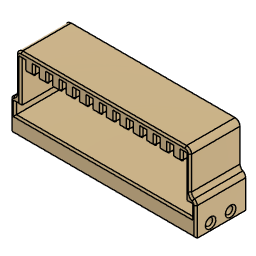
Suporte calha muitos watts 2 v3 (Autodesk Fusion 360 design; units mm, degrees)
Autodesk Fusion 360 part; units mm, degrees
sketch "Sketch1" plane through (0, 0, 0) normal (0, 1, 0) x (1, 0, 0)
  line L0 (0, 0) -> (105, 0)
  line L1 (105, 0) -> (105, -6)
  line L2 (0, -6) -> (0, 0)
  line L3 (51.7, -6) -> (51.7, -31.6)
  line L4 (51.7, -31.6) -> (53.3, -31.6)
  line L5 (53.3, -31.6) -> (53.3, -6)
  line L6 (52.5, -31.6) -> (52.5, 0) construction
  line L7 (3.4, -6) -> (3.4, -31.6)
  line L8 (3.4, -31.6) -> (5, -31.6)
  line L9 (5, -31.6) -> (5, -6)
  line L10 (11.45, -6) -> (11.45, -31.6)
  line L11 (11.45, -31.6) -> (13.05, -31.6)
  line L12 (13.05, -31.6) -> (13.05, -6)
  line L13 (19.5, -6) -> (19.5, -31.6)
  line L14 (19.5, -31.6) -> (21.1, -31.6)
  line L15 (21.1, -31.6) -> (21.1, -6)
  line L16 (27.55, -6) -> (27.55, -31.6)
  line L17 (27.55, -31.6) -> (29.15, -31.6)
  line L18 (29.15, -31.6) -> (29.15, -6)
  line L19 (35.6, -6) -> (35.6, -31.6)
  line L20 (35.6, -31.6) -> (37.2, -31.6)
  line L21 (37.2, -31.6) -> (37.2, -6)
  line L22 (43.65, -6) -> (43.65, -31.6)
  line L23 (43.65, -31.6) -> (45.25, -31.6)
  line L24 (45.25, -31.6) -> (45.25, -6)
  line L25 (59.75, -6) -> (59.75, -31.6)
  line L26 (59.75, -31.6) -> (61.35, -31.6)
  line L27 (61.35, -31.6) -> (61.35, -6)
  line L28 (67.8, -6) -> (67.8, -31.6)
  line L29 (67.8, -31.6) -> (69.4, -31.6)
  line L30 (69.4, -31.6) -> (69.4, -6)
  line L31 (75.85, -6) -> (75.85, -31.6)
  line L32 (75.85, -31.6) -> (77.45, -31.6)
  line L33 (77.45, -31.6) -> (77.45, -6)
  line L34 (83.9, -6) -> (83.9, -31.6)
  line L35 (83.9, -31.6) -> (85.5, -31.6)
  line L36 (85.5, -31.6) -> (85.5, -6)
  line L37 (91.95, -6) -> (91.95, -31.6)
  line L38 (91.95, -31.6) -> (93.55, -31.6)
  line L39 (93.55, -31.6) -> (93.55, -6)
  line L40 (100, -6) -> (100, -31.6)
  line L41 (100, -31.6) -> (101.6, -31.6)
  line L42 (101.6, -31.6) -> (101.6, -6)
  line L43 (11.45, -6) -> (5, -6)
  line L44 (19.5, -6) -> (13.05, -6)
  line L45 (27.55, -6) -> (21.1, -6)
  line L46 (35.6, -6) -> (29.15, -6)
  line L47 (51.7, -6) -> (45.25, -6)
  line L48 (43.65, -6) -> (37.2, -6)
  line L49 (3.4, -6) -> (0, -6)
  line L50 (59.75, -6) -> (53.3, -6)
  line L51 (67.8, -6) -> (61.35, -6)
  line L52 (105, -6) -> (101.6, -6)
  line L53 (100, -6) -> (93.55, -6)
  line L54 (83.9, -6) -> (77.45, -6)
  line L55 (91.95, -6) -> (85.5, -6)
  line L56 (75.85, -6) -> (69.4, -6)
  line L57 (21.4, -31.9) -> (21.4, -6.3)
  line L58 (27.25, -6.3) -> (21.4, -6.3)
  line L59 (27.25, -6.3) -> (27.25, -31.9)
  line L60 (27.25, -31.9) -> (29.45, -31.9)
  line L61 (29.45, -31.9) -> (29.45, -6.3)
  line L62 (35.3, -6.3) -> (29.45, -6.3)
  line L63 (35.3, -6.3) -> (35.3, -31.9)
  line L64 (35.3, -31.9) -> (37.5, -31.9)
  line L65 (37.5, -31.9) -> (37.5, -6.3)
  line L66 (43.35, -6.3) -> (37.5, -6.3)
  line L67 (43.35, -6.3) -> (43.35, -31.9)
  line L68 (43.35, -31.9) -> (45.55, -31.9)
  line L69 (45.55, -31.9) -> (45.55, -6.3)
  line L70 (51.4, -6.3) -> (45.55, -6.3)
  line L71 (51.4, -6.3) -> (51.4, -31.9)
  line L72 (51.4, -31.9) -> (53.6, -31.9)
  line L73 (53.6, -31.9) -> (53.6, -6.3)
  line L74 (59.45, -6.3) -> (53.6, -6.3)
  line L75 (59.45, -6.3) -> (59.45, -31.9)
  line L76 (59.45, -31.9) -> (61.65, -31.9)
  line L77 (61.65, -31.9) -> (61.65, -6.3)
  line L78 (67.5, -6.3) -> (61.65, -6.3)
  line L79 (67.5, -6.3) -> (67.5, -31.9)
  line L80 (67.5, -31.9) -> (69.7, -31.9)
  line L81 (69.7, -31.9) -> (69.7, -6.3)
  line L82 (75.55, -6.3) -> (69.7, -6.3)
  line L83 (75.55, -6.3) -> (75.55, -31.9)
  line L84 (75.55, -31.9) -> (77.75, -31.9)
  line L85 (77.75, -31.9) -> (77.75, -6.3)
  line L86 (83.6, -6.3) -> (77.75, -6.3)
  line L87 (83.6, -6.3) -> (83.6, -31.9)
  line L88 (83.6, -31.9) -> (85.8, -31.9)
  line L89 (85.8, -31.9) -> (85.8, -6.3)
  line L90 (91.65, -6.3) -> (85.8, -6.3)
  line L91 (91.65, -6.3) -> (91.65, -31.9)
  line L92 (91.65, -31.9) -> (93.85, -31.9)
  line L93 (93.85, -31.9) -> (93.85, -6.3)
  line L94 (99.7, -6.3) -> (93.85, -6.3)
  line L95 (99.7, -6.3) -> (99.7, -31.9)
  line L96 (99.7, -31.9) -> (101.9, -31.9)
  line L97 (101.9, -31.9) -> (101.9, -6.3)
  line L98 (105.3, -6.3) -> (101.9, -6.3)
  line L99 (105.3, 0.3) -> (105.3, -6.3)
  line L100 (-0.3, 0.3) -> (105.3, 0.3)
  line L101 (-0.3, -6.3) -> (-0.3, 0.3)
  line L102 (3.1, -6.3) -> (-0.3, -6.3)
  line L103 (3.1, -6.3) -> (3.1, -31.9)
  line L104 (3.1, -31.9) -> (5.3, -31.9)
  line L105 (5.3, -31.9) -> (5.3, -6.3)
  line L106 (11.15, -6.3) -> (5.3, -6.3)
  line L107 (11.15, -6.3) -> (11.15, -31.9)
  line L108 (11.15, -31.9) -> (13.35, -31.9)
  line L109 (13.35, -31.9) -> (13.35, -6.3)
  line L110 (19.2, -6.3) -> (13.35, -6.3)
  line L111 (19.2, -6.3) -> (19.2, -31.9)
  line L112 (19.2, -31.9) -> (21.4, -31.9)
  line L113 (32.15, -34.6) -> (32.15, -9)
  line L114 (32.6, -9) -> (32.15, -9)
  line L115 (32.6, -9) -> (32.6, -34.6)
  line L116 (32.6, -34.6) -> (40.2, -34.6)
  line L117 (40.2, -34.6) -> (40.2, -9)
  line L118 (40.65, -9) -> (40.2, -9)
  line L119 (40.65, -9) -> (40.65, -34.6)
  line L120 (40.65, -34.6) -> (48.25, -34.6)
  line L121 (48.25, -34.6) -> (48.25, -9)
  line L122 (48.7, -9) -> (48.25, -9)
  line L123 (48.7, -9) -> (48.7, -34.6)
  line L124 (48.7, -34.6) -> (56.3, -34.6)
  line L125 (56.3, -34.6) -> (56.3, -9)
  line L126 (56.75, -9) -> (56.3, -9)
  line L127 (56.75, -9) -> (56.75, -34.6)
  line L128 (56.75, -34.6) -> (64.35, -34.6)
  line L129 (64.35, -34.6) -> (64.35, -9)
  line L130 (64.8, -9) -> (64.35, -9)
  line L131 (64.8, -9) -> (64.8, -34.6)
  line L132 (64.8, -34.6) -> (72.4, -34.6)
  line L133 (72.4, -34.6) -> (72.4, -9)
  line L134 (72.85, -9) -> (72.4, -9)
  line L135 (72.85, -9) -> (72.85, -34.6)
  line L136 (72.85, -34.6) -> (80.45, -34.6)
  line L137 (80.45, -34.6) -> (80.45, -9)
  line L138 (80.9, -9) -> (80.45, -9)
  line L139 (80.9, -9) -> (80.9, -34.6)
  line L140 (80.9, -34.6) -> (88.5, -34.6)
  line L141 (88.5, -34.6) -> (88.5, -9)
  line L142 (88.95, -9) -> (88.5, -9)
  line L143 (88.95, -9) -> (88.95, -34.6)
  line L144 (88.95, -34.6) -> (96.55, -34.6)
  line L145 (96.55, -34.6) -> (96.55, -9)
  line L146 (97, -9) -> (96.55, -9)
  line L147 (97, -9) -> (97, -34.6)
  line L148 (97, -34.6) -> (104.6, -34.6)
  line L149 (104.6, -34.6) -> (104.6, -9)
  line L150 (108, -9) -> (104.6, -9)
  line L151 (108, 3) -> (108, -9)
  line L152 (-3, 3) -> (108, 3)
  line L153 (-3, -9) -> (-3, 3)
  line L154 (0.4, -9) -> (-3, -9)
  line L155 (0.4, -9) -> (0.4, -34.6)
  line L156 (0.4, -34.6) -> (8, -34.6)
  line L157 (8, -34.6) -> (8, -9)
  line L158 (8.45, -9) -> (8, -9)
  line L159 (8.45, -9) -> (8.45, -34.6)
  line L160 (8.45, -34.6) -> (16.05, -34.6)
  line L161 (16.05, -34.6) -> (16.05, -9)
  line L162 (16.5, -9) -> (16.05, -9)
  line L163 (16.5, -9) -> (16.5, -34.6)
  line L164 (16.5, -34.6) -> (24.1, -34.6)
  line L165 (24.1, -34.6) -> (24.1, -9)
  line L166 (24.55, -9) -> (24.1, -9)
  line L167 (24.55, -9) -> (24.55, -34.6)
  line L168 (24.55, -34.6) -> (32.15, -34.6)
  line L169 (8, -34.6) -> (97, -34.6)
  line L170 (-3, 3) -> (-3, 10.3)
  line L171 (-3, 10.3) -> (108, 10.3)
  line L172 (108, 10.3) -> (108, 3)
  dimension "d1" = 105
  dimension "d2" = 6
  dimension "d3" = 1.6
  dimension "d4" = 25.6
  dimension "d7" = 8.05
  dimension "d8" = 0
  dimension "d9" = 98.2
  dimension "d10" = -0.3
  dimension "d11" = -3
  dimension "d51" = 10
  constraint horizontal L0
  constraint vertical L1
  constraint horizontal L52
  constraint vertical L2
  constraint coincident L0.start L2.end
  constraint perpendicular L3 L52
  constraint perpendicular L3 L4
  constraint coincident L5.end L52
  constraint perpendicular L5 L52
  constraint midpoint L4 L6.start
  constraint vertical L6
  constraint midpoint L0 L6.end
  constraint horizontal L49
  constraint horizontal L43
  constraint perpendicular L147 L169
  constraint perpendicular L152 L170
  constraint perpendicular L151 L171
  constraint perpendicular L152 L172
  measures "d1" distance of L0.start L0.end
  measures "d2" distance of L0.start L2.start
  measures "d3" distance of L3.end L4.end
  measures "d4" distance of L4.end L5.end
  measures "d9" distance of L7 L42
  measures "d51" distance of L100 L171
extrude "Extrude1" add sketch "Sketch1" along normal blind 30 contours L113 L114 L115 L116 L117 L118 L119 L120 L121 L122 L123 L124 L125 L126 L127 L128 L129 L130 L131 L132 L133 L134 L135 L136 L137 L138 L139 L140 L141 L142 L143 L144 L145 L146 L147 L148 L149 L150 L151 L152 L153 L154 L155 L156 L157 L158 L159 L160 L161 L162 L163 L164 L165 L166 L167 L168 L169 | L113 L114 L115 L169 | L165 L166 L167 L169 | L117 L118 L119 L169 | L161 L162 L163 L169 | L121 L122 L123 L169 | L157 L158 L159 L169 | L125 L126 L127 L169 | L129 L130 L131 L169 | L152 L170 L171 L172 | L133 L134 L135 L169 | L137 L138 L139 L169 | L141 L142 L143 L169 | L145 L146 L147 L169
extrude "Extrude9" cut 12 faces at (9.2, 20, 6.3) (17.25, 20, 6.3) (25.3, 10, 6.3) (33.35, 10, 6.3) (41.4, 10, 6.3) (49.45, 10, 6.3) (57.5, 10, 6.3) (97.75, 10, 6.3) (89.7, 10, 6.3) (81.65, 10, 6.3) (73.6, 10, 6.3) (65.55, 10, 6.3) along direction (0, 0, 1) blind 19
fillet "Fillet7" radius 1 24 edges at (5.3, 15, 25.3) (11.15, 15, 25.3) (13.35, 15, 25.3) (19.2, 15, 25.3) (21.4, 15, 25.3) (27.25, 15, 25.3) (29.45, 15, 25.3) (35.3, 15, 25.3) (37.5, 15, 25.3) (43.35, 15, 25.3) (45.55, 15, 25.3) (51.4, 15, 25.3) (53.6, 15, 25.3) (59.45, 15, 25.3) (61.65, 15, 25.3) (67.5, 15, 25.3) (69.7, 15, 25.3) (75.55, 15, 25.3) (77.75, 15, 25.3) (83.6, 15, 25.3) (91.65, 15, 25.3) (85.8, 15, 25.3) (99.7, 15, 25.3) (93.85, 15, 25.3)
chamfer "Chamfer4" distance 1 angle 45 120 edges at (5.3, 0, 29.1) (11.15, 0, 29.1) (10.8571, 0, 25.5929) (8.225, 0, 25.3) (5.5929, 0, 25.5929) (13.35, 0, 29.1) (19.2, 0, 29.1) (18.9071, 0, 25.5929) (16.275, 0, 25.3) (13.6429, 0, 25.5929) (21.4, 0, 29.1) (27.25, 0, 29.1) (26.9571, 0, 25.5929) (24.325, 0, 25.3) (21.6929, 0, 25.5929) (29.45, 0, 29.1) (35.3, 0, 29.1) (35.0071, 0, 25.5929) (32.375, 0, 25.3) (29.7429, 0, 25.5929) (37.5, 0, 29.1) (43.35, 0, 29.1) (43.0571, 0, 25.5929) (40.425, 0, 25.3) (37.7929, 0, 25.5929) (45.55, 0, 29.1) (51.4, 0, 29.1) (51.1071, 0, 25.5929) (48.475, 0, 25.3) (45.8429, 0, 25.5929) (59.45, 0, 29.1) (59.1571, 0, 25.5929) (56.525, 0, 25.3) (53.8929, 0, 25.5929) (53.6, 0, 29.1) (61.65, 0, 29.1) (67.5, 0, 29.1) (67.2071, 0, 25.5929) (64.575, 0, 25.3) (61.9429, 0, 25.5929) (69.7, 0, 29.1) (75.55, 0, 29.1) (75.2571, 0, 25.5929) (72.625, 0, 25.3) (69.9929, 0, 25.5929) (99.7, 0, 29.1) (99.4071, 0, 25.5929) (96.775, 0, 25.3) (94.1429, 0, 25.5929) (93.85, 0, 29.1) (91.65, 0, 29.1) (91.3571, 0, 25.5929) (88.725, 0, 25.3) (86.0929, 0, 25.5929) (85.8, 0, 29.1) (83.6, 0, 29.1) (83.3071, 0, 25.5929) (80.675, 0, 25.3) (78.0429, 0, 25.5929) (77.75, 0, 29.1) (99.7, 30, 29.1) (99.4071, 30, 25.5929) (96.775, 30, 25.3) (94.1429, 30, 25.5929) (93.85, 30, 29.1) (72.625, 30, 25.3) (69.9929, 30, 25.5929) (69.7, 30, 29.1) (75.55, 30, 29.1) (75.2571, 30, 25.5929) (88.725, 30, 25.3) (86.0929, 30, 25.5929) (85.8, 30, 29.1) (91.65, 30, 29.1) (91.3571, 30, 25.5929) (80.675, 30, 25.3) (78.0429, 30, 25.5929) (77.75, 30, 29.1) (83.6, 30, 29.1) (83.3071, 30, 25.5929) (64.575, 30, 25.3) (61.9429, 30, 25.5929) (61.65, 30, 29.1) (67.5, 30, 29.1) (67.2071, 30, 25.5929) (56.525, 30, 25.3) (53.8929, 30, 25.5929) (53.6, 30, 29.1) (59.45, 30, 29.1) (59.1571, 30, 25.5929) (48.475, 30, 25.3) (45.8429, 30, 25.5929) (45.55, 30, 29.1) (51.4, 30, 29.1) (51.1071, 30, 25.5929) (40.425, 30, 25.3) (37.7929, 30, 25.5929) (37.5, 30, 29.1) (43.35, 30, 29.1) (43.0571, 30, 25.5929) (35.0071, 30, 25.5929) (35.3, 30, 29.1) (29.45, 30, 29.1) (29.7429, 30, 25.5929) (32.375, 30, 25.3) (24.325, 30, 25.3) (21.6929, 30, 25.5929) (21.4, 30, 29.1) (27.25, 30, 29.1) (26.9571, 30, 25.5929) (16.275, 30, 25.3) (13.6429, 30, 25.5929) (13.35, 30, 29.1) (19.2, 30, 29.1) (18.9071, 30, 25.5929) (10.8571, 30, 25.5929) (11.15, 30, 29.1) (5.3, 30, 29.1) (5.5929, 30, 25.5929) (8.225, 30, 25.3)
fillet "Fillet8" radius 3 6 edges at (104.6, 15, 9) (108, 15, 9) (-3, 15, 9) (0.4, 15, 9) (0.4, 15, 34.6) (104.6, 15, 34.6)
sketch "Sketch6" plane through (108, 0, 0) normal (1, 0, 0) x (0, 1, 0)
  line L0 (30, 6.5926) -> (0, 6.5926)
  line L1 (0, 6.5926) -> (0, -10.3)
  line L2 (0, -10.3) -> (30, -10.3)
  line L3 (30, -10.3) -> (30, 6.5926)
  circle A0 centre (9, -6.3) radius 2.15
  circle A1 centre (21, -6.3) radius 2.15
  line L4 (9, -6.3) -> (21, -6.3) construction
  line L5 (15, -6.3) -> (15, -10.3) construction
  dimension "d59" = 4.3
  dimension "d60" = 12
  dimension "d61" = 4
  constraint equal A0 A1
  constraint coincident A0.centre L4.start
  constraint coincident A1.centre L4.end
  constraint horizontal L4
  constraint midpoint L4 L5.start
  constraint midpoint L2 L5.end
  constraint vertical L5
  measures "d59" diameter of A1
  measures "d60" distance of A0.centre A1.centre
  measures "d61" distance of L5.start L5.end
extrude "Extrude10" cut sketch "Sketch6" against normal blind 176 contours A0 | A1
chamfer "Chamfer5" distance 1 angle 45 4 edges at (108, 18.9955, -5.5225) (108, 6.9955, -5.5225) (-3, 6.9955, -7.0775) (-3, 18.9955, -7.0775)
chamfer "Chamfer6" distance 1 angle 45 26 edges at (104.6, 0, 21.8) (105.0603, 0, 10.4031) (107.5397, 0, 8.1895) (108, 0, -1.8537) (-3, 0, -1.8537) (-2.5397, 0, 8.1895) (-0.0603, 0, 10.4031) (0.4, 0, 21.8) (1.2787, 0, 33.7213) (52.5, 0, 34.6) (103.7213, 0, 33.7213) (52.5, 0, -10.3) (3.1, 0, 19.1) (-0.3, 0, 3) (52.5, 0, -0.3) (1.4, 0, 6.3) (101.9, 0, 19.1) (103.6, 0, 6.3) (105.3, 0, 3) (101.9, 30, 19.1) (103.6, 30, 6.3) (105.3, 30, 3) (52.5, 30, -0.3) (-0.3, 30, 3) (1.4, 30, 6.3) (3.1, 30, 19.1)
equation "d7 = 6.55 mm + 1.5 mm"
named bodies: "Lateral A"
